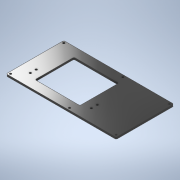
# Autodesk Inventor part: Sole_frame
Saved by Autodesk Inventor 2020.4 (Build 244396000, 396)
## iProperties
Part Number: Sole_frame
Material: GFRP
Document SubType Name: Modeling
Designer: Masato Kubotera
Density: 1.75 g/cm^3
Appearance: 低 光沢 - 黒
Description: GFRP T3
Mass: 61.6656 g
Surface Area: 261.936 cm^2
Volume: 35.2375 cm^3
Author: Masato Kubotera
Autodesk Inventor part; units mm, degrees
ref_plane "YZ Plane" through (0, 0, 0) normal (1, 0, 0) x (0, 1, 0)
ref_plane "XZ Plane" through (0, 0, 0) normal (0, 1, 0) x (-1, 0, 0)
ref_plane "XY Plane" through (0, 0, 0) normal (0, 0, 1) x (1, 0, 0)
sketch "スケッチ1" plane through (0, 0, 0) normal (0, 0, 1) x (1, 0, 0)
  line L0 (-98.235, 67.25) -> (78.265, 67.25)
  line L1 (78.265, 67.25) -> (78.265, -25.25)
  line L2 (78.265, -25.25) -> (-98.235, -25.25)
  line L3 (-98.235, -25.25) -> (-98.235, 67.25)
  line L4 (-98.235, 67.25) -> (78.265, -25.25) construction
  line L5 (78.265, 67.25) -> (-98.235, -25.25) construction
  line L6 (-98.235, 21) -> (78.265, 21) construction
  line L7 (-98.235, 0) -> (78.265, 0) construction
  line L8 (-80, 4.75) -> (-80, -4.75) construction
  circle A0 centre (-80, -4.75) radius 1.6
  line L9 (0, 67.25) -> (0, -25.25) construction
  line L10 (18, -4.75) -> (18, 4.75) construction
  circle A1 centre (18, -4.75) radius 1.6
  circle A2 centre (-80, 4.75) radius 1.6
  circle A3 centre (18, 4.75) radius 1.6
  line L11 (74.765, -21.75) -> (-94.735, -21.75) construction
  line L12 (-94.735, -21.75) -> (-94.735, 63.75) construction
  line L13 (-94.735, 63.75) -> (74.765, 63.75) construction
  line L14 (74.765, 63.75) -> (74.765, -21.75) construction
  line L15 (74.765, -21.75) -> (-94.735, 63.75) construction
  line L16 (-94.735, -21.75) -> (74.765, 63.75) construction
  circle A4 centre (-94.735, 63.75) radius 1.6
  circle A5 centre (0, 63.75) radius 1.6
  circle A6 centre (74.765, 63.75) radius 1.6
  circle A7 centre (-94.735, -21.75) radius 1.6
  circle A8 centre (0, -21.75) radius 1.6
  circle A9 centre (74.765, -21.75) radius 1.6
  line L17 (15, 12.5) -> (21, 12.5) construction
  line L18 (21, 12.5) -> (21, -12.5) construction
  line L19 (21, -12.5) -> (15, -12.5) construction
  line L20 (15, -12.5) -> (15, 12.5) construction
  line L21 (15, 12.5) -> (21, -12.5) construction
  line L22 (21, 12.5) -> (15, -12.5) construction
  line L23 (-83, 12.5) -> (-77, 12.5) construction
  line L24 (-77, 12.5) -> (-77, -12.5) construction
  line L25 (-77, -12.5) -> (-83, -12.5) construction
  line L26 (-83, -12.5) -> (-83, 12.5) construction
  line L27 (-83, 12.5) -> (-77, -12.5) construction
  line L28 (-77, 12.5) -> (-83, -12.5) construction
  line L29 (-67, 52.25) -> (5, 52.25)
  line L30 (5, 52.25) -> (5, -10.25)
  line L31 (5, -10.25) -> (-67, -10.25)
  line L32 (-67, -10.25) -> (-67, 52.25)
  line L33 (-67, 52.25) -> (5, -10.25) construction
  line L34 (5, 52.25) -> (-67, -10.25) construction
  point P0 (0, 0)
  point P1 (-9.985, 21)
  point P2 (-80, 0)
  point P3 (18, 0)
  point P4 (-31, 21)
  dimension "d0" = 176.5
  dimension "d1" = 92.5
  dimension "d2" = 25.25
  dimension "d3" = 3.2
  dimension "d4" = 9.5
  dimension "d5" = 9.5
  dimension "d6" = 3.2
  dimension "d9" = 3.5
  dimension "d10" = 3.5
  dimension "d11" = 3.2
  dimension "d13" = 3.2
  dimension "d15" = 3.2
  dimension "d16" = 78.265
  dimension "d17" = 6
  dimension "d18" = 25
  dimension "d19" = 21
  dimension "d20" = 6
  dimension "d21" = 25
  dimension "d22" = 104
  dimension "d23" = 15
  dimension "d24" = 15
  dimension "d25" = 10
  dimension "d26" = 10
  constraints: 70 end point, 14 midpoint, 10 centre point, 10 parallel, 10 point on line, 7 perpendicular, 5 horizontal, 5 symmetric about line, 4 coincident, 2 vertical, 5 other
  measures "d0" distance of L1.end L2.end
  measures "d1" distance of L0.end L1.end
  measures "d2" distance of L2.end L7.start
  measures "d3" diameter of A0
  measures "d4" distance of L8.start L8.end
  measures "d5" distance of L10.start L10.end
  measures "d6" diameter of A1
  measures "d9" horizontal distance of L0.start L12.end
  measures "d10" horizontal distance of L0.start L12.end
  measures "d11" diameter of A4
  measures "d13" diameter of A5
  measures "d15" diameter of A6
  measures "d16" distance of L0.end L9.start
  measures "d17" distance of L18.end L19.end
  measures "d18" distance of L17.end L18.end
  measures "d19" horizontal distance of L17.end point (0, 0)
  measures "d20" distance of L24.end L25.end
  measures "d21" distance of L23.end L24.end
  measures "d22" distance of L18.end L25.end
  measures "d23" distance between parallel lines of L29 L0
  measures "d24" distance between parallel lines of L2 L31
  measures "d25" distance between parallel lines of L32 L24
  measures "d26" distance between parallel lines of L20 L30
extrude "押し出し1" add sketch "スケッチ1" along normal blind 3
fillet "フィレット1" radius 2 4 edges at (-98.235, 67.25, 1.5) (78.265, 67.25, 1.5) (78.265, -25.25, 1.5) (-98.235, -25.25, 1.5)
fillet "フィレット2" radius 2 4 edges at (-67, 52.25, 1.5) (-67, -10.25, 1.5) (5, -10.25, 1.5) (5, 52.25, 1.5)
equation "\"d3\" = d6"
equation "\"d4\" = d5"
equation "\"d10\" = d9"
equation "\"d11\" = d3"
equation "\"d13\" = d11"
equation "\"d15\" = d13"
equation "\"d20\" = d17"
equation "\"d21\" = d18"
